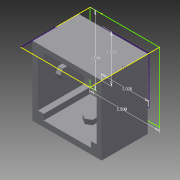
# Autodesk Inventor part: freeholder
Saved by Autodesk Inventor 2013 SP2 (Build 170200200, 200)
## iProperties
Created: 2015-05-11
Part Number: freeholder
Document SubType Name: Modeling
Designer: 2016ahoganso
Density: 1 g/cm^3
Material: Generic
Author: 2016ahoganso
Autodesk Inventor part; units mm, degrees
ref_plane "YZ Plane" through (0, 0, 0) normal (1, 0, 0) x (0, 1, 0)
ref_plane "XZ Plane" through (0, 0, 0) normal (0, 1, 0) x (-1, 0, 0)
ref_plane "XY Plane" through (0, 0, 0) normal (0, 0, 1) x (1, 0, 0)
sketch "Sketch1" plane through (0, 0, 0) normal (0, 0, 1) x (1, 0, 0)
  line L0 (0, 0) -> (25.908, 0)
  line L1 (25.908, 0) -> (25.908, 25.908)
  line L2 (25.908, 25.908) -> (0, 25.908)
  line L3 (0, 25.908) -> (0, 0)
  line L4 (-6.35, 0) -> (-6.35, -6.35)
  line L5 (-6.35, -6.35) -> (0, -6.35)
  line L6 (-6.35, -6.35) -> (31.75, -6.35)
  line L7 (31.75, -6.35) -> (31.75, 31.75)
  line L8 (31.75, 31.75) -> (-6.35, 31.75)
  line L9 (-6.35, 31.75) -> (-6.35, -6.35)
  dimension "d0" = 25.908
  dimension "d1" = 25.908
  dimension "d4" = 38.1
  dimension "d5" = 38.1
  constraints: 20 end point, 4 parallel, 2 horizontal, 2 perpendicular
  measures "d0" distance of L0.start L0.end
  measures "d1" distance of L2.end L0.start
  measures "d4" distance of L4.end L6.end
  measures "d5" distance of L8.end L4.end
extrude "Extrusion1" add sketch "Sketch1" along normal blind 38.1
sketch "Sketch2" plane through (-6.35, 31.75, 0) normal (0, 1, 0) x (1, 0, 0)
  line L0 (0, -38.1) -> (38.1, -38.1) projected
  line L1 (38.1, 0) -> (38.1, -38.1) projected
  line L2 (38.1, 0) -> (0, 0) projected
  line L3 (0, 0) -> (0, -38.1) projected
  line L4 (0, -38.1) -> (0, -19.05)
  line L5 (0, 0) -> (0, -38.1) projected
  point P0 (6.35, 0)
  constraints: 2 end point, 1 coincident, 1 midpoint
sketch "Sketch3" plane through (-6.35, 31.75, 0) normal (0, 1, 0) x (1, 0, 0)
  line L0 (0, -38.1) -> (38.1, -38.1) projected
  line L1 (38.1, 0) -> (38.1, -38.1) projected
  line L2 (38.1, 0) -> (0, 0) projected
  line L3 (0, 0) -> (0, -38.1) projected
  point P0 (6.35, 0)
  point P1 (38.1, -19.05)
  constraints: 1 midpoint
sketch "Sketch4" plane through (0, 0, 38.1) normal (0, 0, 1) x (1, 0, 0)
  line L0 (0, 0) -> (25.908, 0)
  line L1 (25.908, 0) -> (25.908, -3.175)
  line L2 (25.908, -3.175) -> (0, -3.175)
  line L3 (0, -3.175) -> (0, 0)
  line L4 (25.908, 0) -> (29.083, 0)
  line L5 (29.083, 0) -> (29.083, 25.908)
  line L6 (29.083, 25.908) -> (25.908, 25.908)
  line L7 (25.908, 25.908) -> (25.908, 0)
  line L8 (25.908, 25.908) -> (0, 25.908)
  line L9 (0, 25.908) -> (0, 29.083)
  line L10 (0, 29.083) -> (25.908, 29.083)
  line L11 (25.908, 29.083) -> (25.908, 25.908)
  line L12 (0, 0) -> (-3.175, 0)
  line L13 (-3.175, 0) -> (-3.175, 25.908)
  line L14 (-3.175, 25.908) -> (0, 25.908)
  line L15 (0, 25.908) -> (0, 0)
  dimension "d8" = 3.175
  dimension "d9" = 3.175
  dimension "d10" = 3.175
  dimension "d11" = 3.175
  constraints: 32 end point, 8 parallel, 4 horizontal, 4 perpendicular
  measures "d8" distance of L0.end L1.end
  measures "d9" distance of L6.end L5.end
  measures "d10" distance of L8.end L9.end
  measures "d11" distance of L13.end L14.end
extrude "Extrusion2" cut sketch "Sketch4" against normal blind 38.1 contours L0 L1 L2 L3 | L12 L13 L14 L15 | L7 L6 L5 L4 | L9 L10 L11 L8
sketch "Sketch5" plane through (0, 29.083, 38.1) normal (0, -1, 0) x (1, 0, 0)
  line L0 (0, 0) -> (0, -38.1) projected
  line L1 (0, 0) -> (0, -19.05)
  line L2 (0, -19.05) -> (12.954, -19.05)
  line L3 (25.908, 0) -> (25.908, -38.1) projected
  line L4 (12.954, -19.05) -> (12.954, -15.9258)
  line L5 (12.954, -15.9258) -> (15.6596, -17.4879)
  line L6 (15.6596, -17.4879) -> (15.6596, -20.6121)
  line L7 (15.6596, -20.6121) -> (12.954, -22.1742)
  line L8 (12.954, -22.1742) -> (10.2484, -20.6121)
  line L9 (10.2484, -20.6121) -> (10.2484, -17.4879)
  line L10 (10.2484, -17.4879) -> (12.954, -15.9258)
  dimension "d14" = 19.05
  dimension "d22" = 3.1242
  constraints: 18 end point, 2 coincident, 1 midpoint, 1 parallel, 1 perpendicular, 13 other
  measures "d14" distance of L0.start L1.end
  measures "d22" distance of L4.start L4.end
extrude "Extrusion3" add sketch "Sketch5" along normal blind 2.54
sketch "Sketch6" plane through (-3.175, 0, 38.1) normal (1, 0, 0) x (0, 0, -1)
  line L0 (38.1, 25.908) -> (38.1, 0) projected
  line L1 (38.1, 0) -> (38.1, 12.954)
  line L2 (38.1, 12.954) -> (19.05, 12.954)
  line L3 (19.05, 12.954) -> (22.1742, 12.954)
  line L4 (22.1742, 12.954) -> (20.6121, 10.2484)
  line L5 (20.6121, 10.2484) -> (17.4879, 10.2484)
  line L6 (17.4879, 10.2484) -> (15.9258, 12.954)
  line L7 (15.9258, 12.954) -> (17.4879, 15.6596)
  line L8 (17.4879, 15.6596) -> (20.6121, 15.6596)
  line L9 (20.6121, 15.6596) -> (22.1742, 12.954)
  dimension "d19" = 12.954
  dimension "d20" = 19.05
  dimension "d23" = 3.1242
  constraints: 18 end point, 1 coincident, 1 midpoint, 1 perpendicular, 1 point on line, 13 other
  measures "d19" distance of L0.end L1.end
  measures "d20" distance of L1.end L2.end
  measures "d23" distance of L2.end L3.end
extrude "Extrusion4" add sketch "Sketch6" along normal blind 2.54
sketch "Sketch7" plane through (0, -3.175, 38.1) normal (0, 1, 0) x (1, 0, 0)
  line L0 (0, 0) -> (0, 38.1) projected
  line L1 (0, 0) -> (0, 19.05)
  line L2 (0, 19.05) -> (12.954, 19.05)
  line L3 (12.954, 19.05) -> (12.954, 15.9258)
  line L4 (12.954, 15.9258) -> (10.2484, 17.4879)
  line L5 (10.2484, 17.4879) -> (10.2484, 20.6121)
  line L6 (10.2484, 20.6121) -> (12.954, 22.1742)
  line L7 (12.954, 22.1742) -> (15.6596, 20.6121)
  line L8 (15.6596, 20.6121) -> (15.6596, 17.4879)
  line L9 (15.6596, 17.4879) -> (12.954, 15.9258)
  dimension "d26" = 19.05
  dimension "d27" = 12.954
  dimension "d28" = 3.1242
  constraints: 18 end point, 1 coincident, 1 midpoint, 1 parallel, 1 perpendicular, 13 other
  measures "d26" distance of L0.start L1.end
  measures "d27" distance of L1.end L2.end
  measures "d28" distance of L2.end L3.end
extrude "Extrusion5" add sketch "Sketch7" along normal blind 2.54
sketch "Sketch8" plane through (29.083, 0, 38.1) normal (-1, 0, 0) x (0, 0, 1)
  line L0 (0, 0) -> (-19.05, 0)
  line L1 (-38.1, 0) -> (0, 0) projected
  line L2 (-19.05, 0) -> (-19.05, 12.954)
  line L3 (-19.05, 12.954) -> (-15.9258, 12.954)
  line L4 (-15.9258, 12.954) -> (-17.4879, 10.2484)
  line L5 (-17.4879, 10.2484) -> (-20.6121, 10.2484)
  line L6 (-20.6121, 10.2484) -> (-22.1742, 12.954)
  line L7 (-22.1742, 12.954) -> (-20.6121, 15.6596)
  line L8 (-20.6121, 15.6596) -> (-17.4879, 15.6596)
  line L9 (-17.4879, 15.6596) -> (-15.9258, 12.954)
  dimension "d31" = 19.05
  dimension "d32" = 12.954
  dimension "d33" = 3.1242
  constraints: 18 end point, 2 perpendicular, 1 coincident, 1 midpoint, 13 other
  measures "d31" distance of L0.start L0.end
  measures "d32" distance of L0.end L2.end
  measures "d33" distance of L2.end L3.end
extrude "Extrusion6" add sketch "Sketch8" along normal blind 2.54
sketch "Sketch9" plane through (0, 0, 38.1) normal (0, 0, 1) x (1, 0, 0)
  line L0 (0, 25.908) -> (0, 29.083) projected
  line L1 (0, 29.083) -> (25.908, 29.083) projected
  line L2 (25.908, 29.083) -> (25.908, 25.908) projected
  line L3 (25.908, 25.908) -> (29.083, 25.908) projected
  line L4 (29.083, 25.908) -> (29.083, 0) projected
  line L5 (29.083, 0) -> (25.908, 0) projected
  line L6 (25.908, 0) -> (25.908, -3.175) projected
  line L7 (25.908, -3.175) -> (0, -3.175) projected
  line L8 (0, -3.175) -> (0, 0) projected
  line L9 (0, 0) -> (-3.175, 0) projected
  line L10 (-3.175, 0) -> (-3.175, 25.908) projected
  line L11 (-3.175, 25.908) -> (0, 25.908) projected
  line L12 (-6.35, -6.35) -> (-6.35, 31.75) projected
  line L13 (31.75, -6.35) -> (-6.35, -6.35) projected
  line L14 (31.75, 31.75) -> (31.75, -6.35) projected
  line L15 (-6.35, 31.75) -> (31.75, 31.75) projected
extrude "Extrusion7" cut sketch "Sketch9" against normal blind 6.35
extrude "Extrusion8" cut sketch "Sketch1" along normal blind 6.35
body "Solid1"
